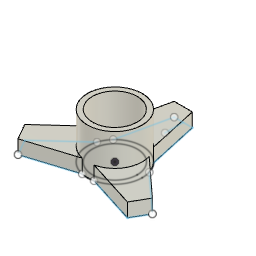
無題 (Autodesk Fusion 360 design; units mm, degrees)
Autodesk Fusion 360 part; units mm, degrees
sketch "スケッチ1" plane through (0, 0, 0) normal (0, 0, 1) x (1, 0, 0)
  circle A0 centre (0, 0) radius 4.9
  circle A1 centre (0, 0) radius 6
  line L0 (-2, 15) -> (2, 15)
  line L1 (2, 15) -> (4.4261, 4.0509)
  line L2 (0, 15) -> (0, 11)
  line L3 (-2, 15) -> (-4.4261, 4.0509)
  line L4 (-13.9904, -5.7679) -> (-5.7212, 1.8076)
  line L5 (-11.9904, -9.2321) -> (-13.9904, -5.7679)
  line L6 (-11.9904, -9.2321) -> (-1.2952, -5.8585)
  line L7 (11.9904, -9.2321) -> (1.2952, -5.8585)
  line L8 (13.9904, -5.7679) -> (11.9904, -9.2321)
  line L9 (13.9904, -5.7679) -> (5.7212, 1.8076)
  dimension "d1" = 9.8
  dimension "d2" = 12
  dimension "d4" = 360
  constraint coincident A0.centre A1.centre
  constraint horizontal L0
  constraint coincident A1 L1.end
  constraint midpoint L0 L2.start
  constraint perpendicular L0 L2
  constraint symmetric L0.end L2 L0.start
  constraint symmetric L1.end L2 L3.end
  measures "d1" diameter of A0
  measures "d2" diameter of A1
extrude "押し出し1" add sketch "スケッチ1" along normal blind 2 contours A0 | A1 | A1 L7 L8 L9 | A1 L0 L1 L3 | A1 L4 L5 L6
extrude "押し出し2" add sketch "スケッチ1" along normal blind 8 from surface at 2 contours A1
move_face "面を移動1" by (0, 0, 1) 3 faces at (10.3743, -6.0305, 2) (-10.3923, -6, 2) (0, 12, 2)
